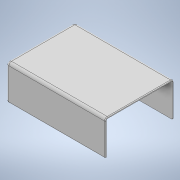
# Autodesk Inventor part: ECG_cover
Saved by Autodesk Inventor 2022 (Build 260153000, 153)
## iProperties
Created: 2021-11-06
Part Number: ECG_cover
Material: Generic
Document SubType Name: Modeling
Designer: Karl
Density: 1 g/cm^3
Appearance: Default
Author: Karl
Autodesk Inventor part; units mm, degrees
ref_plane "YZ Plane" through (0, 0, 0) normal (1, 0, 0) x (0, 1, 0)
ref_plane "XZ Plane" through (0, 0, 0) normal (0, 1, 0) x (-1, 0, 0)
ref_plane "XY Plane" through (0, 0, 0) normal (0, 0, 1) x (1, 0, 0)
sketch "Sketch1" plane through (0, 0, 0) normal (0, 0, 1) x (1, 0, 0)
  line L0 (-47.625, -16.6751) -> (47.625, -16.6751)
  line L1 (47.625, -16.6751) -> (47.625, 16.6751)
  line L2 (47.625, 16.6751) -> (-47.625, 16.6751)
  line L3 (-47.625, 16.6751) -> (-47.625, -16.6751)
  line L4 (-47.625, -16.6751) -> (47.625, 16.6751) construction
  line L5 (47.625, -16.6751) -> (-47.625, 16.6751) construction
  point P0 (0, 0)
  dimension "d0" = 95.25
  dimension "d1" = 33.3502
  constraints: 12 end point, 2 midpoint, 2 parallel, 1 horizontal, 1 perpendicular
  measures "d0" distance of L2.end L1.end
  measures "d1" distance of L1.end L0.end
extrude "Extrusion1" add sketch "Sketch1" along normal blind 66.04
shell "Shell1" thickness 1.27 removed faces 2 at (-15.875, -16.6751, 44.0267) at (47.625, -5.5584, 44.0267)
sketch "Sketch2" plane through (-46.355, -16.6751, 1.27) normal (1, 0, 0) x (0, 0, -1)
  line L0 (0, 32.0802) -> (0, 0) projected
  line L1 (0, 0) -> (-63.5, 0) projected
  circle A0 centre (-14.351, 19.1262) radius 3.2512
  point P0 (1.27, 16.6751)
  dimension "d5" = 14.351
  dimension "d6" = 19.1262
  dimension "d7" = 6.5024
  constraints: 1 centre point, 1 coincident
  measures "d5" distance from line of L0 point (-14.351, 19.126)
  measures "d6" distance from line of L1 point (-14.351, 19.126)
  measures "d7" diameter of A0
extrude "Extrusion2" cut sketch "Sketch2" against normal up to surface (1.27 mm away)
fillet "Fillet1" radius 2.54 5 edges at (0, 16.6751, 66.04) (-47.625, 16.6751, 33.02) (0, 16.6751, 0) (-47.625, 0, 0) (-47.625, 0, 66.04)
fillet "Fillet2" radius 0.635 5 edges at (47.625, -1.27, 0) (47.625, 15.9312, 0.7439) (47.625, 16.6751, 33.02) (47.625, 15.9312, 65.2961) (47.625, -1.27, 66.04)
fillet "Fillet3" radius 0.635 9 edges at (47.439, -16.6751, 65.854) (47.625, -16.6751, 65.0875) (-46.8811, -16.6751, 65.2961) (-47.625, -16.6751, 33.02) (-46.8811, -16.6751, 0.7439) (0.9525, -16.6751, 0) (47.439, -16.6751, 0.186) (47.625, -16.6751, 0.9525) (0.9525, -16.6751, 66.04)
body "Solid1"
